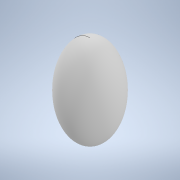
# Autodesk Inventor part: Egg
Saved by Autodesk Inventor 2022 (Build 260153000, 153)
## iProperties
Created: 2022-02-16
Part Number: Egg
Material: Generic
Document SubType Name: Modeling
Designer: Nathan Griffith
Density: 1 g/cm^3
Appearance: Default
Author: Nathan Griffith
Autodesk Inventor part; units mm, degrees
ref_plane "YZ Plane" through (0, 0, 0) normal (1, 0, 0) x (0, 1, 0)
ref_plane "XZ Plane" through (0, 0, 0) normal (0, 1, 0) x (-1, 0, 0)
ref_plane "XY Plane" through (0, 0, 0) normal (0, 0, 1) x (1, 0, 0)
sketch "Sketch1" plane through (0, 0, 0) normal (0, 0, 1) x (1, 0, 0)
  line L0 (0, 31.115) -> (-18.415, 31.115)
  line L1 (-18.415, 31.115) -> (-18.415, -31.115)
  line L2 (-18.415, 31.115) -> (-18.415, -31.115)
  line L3 (-18.415, -31.115) -> (18.415, -31.115)
  line L4 (18.415, -31.115) -> (-18.415, 31.115)
  line L5 (-18.415, -31.115) -> (18.415, 31.115)
  ellipse E0 centre (0, 0) end of major axis (0, 31.115) minor radius 18.415 (0, 31.115) -> (0, -31.115) ccw
  line L6 (0, 31.115) -> (0, -31.115)
  line L7 (-18.415, 0) -> (0, 0)
  line L8 (-18.415, 31.115) -> (18.415, 31.115)
  constraints: 18 end point, 4 other
revolve "Revolution1" add sketch "Sketch1" angle 360 about axis through (0, 31.115, 0) along (0, -1, 0) contours L6 L4 E0 | L4 L7 E0 | L6 E0 L5 | L5 E0 L7
body "Solid1"
